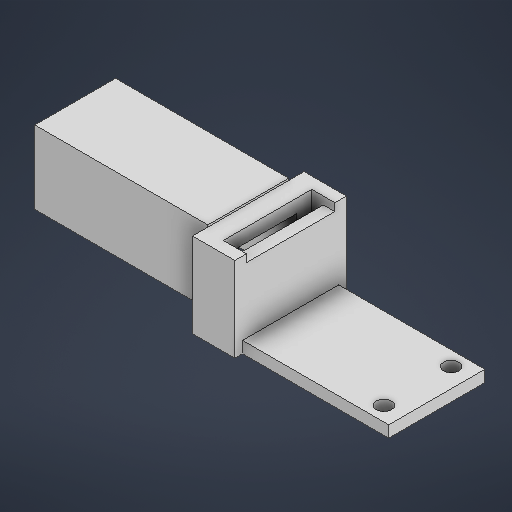
# Autodesk Inventor part: rgb-holder-group2
Saved by Autodesk Inventor 2026.1 (Build 301233000, 233)
## iProperties
Created: 2026-03-11
Part Number: rgb-holder-group2
Material: Generic
Document SubType Name: Modeling
Designer: ba2032
Density: 1 g/cm^3
Appearance: Default
Author: ba2032
Autodesk Inventor part; units mm, degrees
ref_plane "YZ Plane" through (0, 0, 0) normal (1, 0, 0) x (0, 1, 0)
ref_plane "XZ Plane" through (0, 0, 0) normal (0, 1, 0) x (-1, 0, 0)
ref_plane "XY Plane" through (0, 0, 0) normal (0, 0, 1) x (1, 0, 0)
sketch "Sketch1" plane through (0, 0, 0) normal (0, 1, 0) x (-1, 0, 0)
  line L0 (-20, 12.5) -> (20, 12.5)
  line L1 (20, 12.5) -> (20, -12.5)
  line L2 (20, -12.5) -> (-20, -12.5)
  line L3 (-20, -12.5) -> (-20, 12.5)
  line L4 (-20, 12.5) -> (20, -12.5) construction
  line L5 (20, 12.5) -> (-20, -12.5) construction
  circle A0 centre (-15, 8.75) radius 2
  circle A1 centre (-15, -8.75) radius 2
  point P0 (0, 0)
  dimension "d0" = 40
  dimension "d1" = 25
  dimension "d2" = 4
  dimension "d3" = 4
  constraints: 12 end point, 2 centre point, 2 midpoint, 2 parallel, 1 horizontal, 1 perpendicular
  measures "d0" distance of L1.end L2.end
  measures "d1" distance of L0.end L1.end
  measures "d2" diameter of A0
  measures "d3" diameter of A1
extrude "Extrusion1" add sketch "Sketch1" along normal blind 3 contours L0 L1 L2 L3 | A1
extrude "Extrusion2" cut sketch "Sketch1" along normal blind 3 contours A0 | A1
sketch "Sketch3" plane through (-20, 0, -12.5) normal (-1, 0, 0) x (0, 0, 1)
  line L0 (0, 0) -> (25, 0) projected
  line L1 (0, 0) -> (25, 0)
  line L2 (25, 0) -> (25, 22)
  line L3 (25, 22) -> (0, 22)
  line L4 (0, 22) -> (0, 0)
  point P0 (12.5, 0)
  dimension "d14" = 22
  constraints: 8 end point, 2 parallel, 1 horizontal, 1 perpendicular
  measures "d14" distance of L2.end L0.end
extrude "Extrusion4" add sketch "Sketch3" along normal blind 9
sketch "Sketch4" plane through (-20, 22, 12.5) normal (0, 1, 0) x (1, 0, 0)
  line L0 (-4, 24) -> (-1, 24)
  line L1 (-1, 24) -> (-1, 1)
  line L2 (-1, 1) -> (-4, 1)
  line L3 (-4, 1) -> (-4, 24)
  point P0 (20, 12.5)
  dimension "d17" = 3
  dimension "d18" = 23
  constraints: 8 end point, 2 parallel, 1 horizontal, 1 perpendicular
  measures "d17" distance of L0.start L0.end
  measures "d18" distance of L0.end L1.end
extrude "Extrusion5" cut sketch "Sketch4" against normal blind 21
sketch "Sketch6" plane through (-21, 22, -11.5) normal (-1, 0, 0) x (0, 0, 1)
  line L0 (0, 0) -> (23, 0) projected
  line L1 (0, 0) -> (23, 0)
  line L2 (23, 0) -> (23, -2)
  line L3 (23, -2) -> (0, -2)
  line L4 (0, -2) -> (0, 0)
  point P0 (11.5, -22)
  dimension "d26" = 2
  constraints: 8 end point, 2 parallel, 1 horizontal, 1 perpendicular
  measures "d26" distance of L0.end L2.end
extrude "Extrusion7" cut sketch "Sketch6" against normal blind 3
sketch "Sketch5" plane through (-29, 0, -12.5) normal (-1, 0, 0) x (0, 0, 1)
  line L0 (20, 18.5) -> (20, 3.5)
  line L1 (20, 3.5) -> (5, 3.5)
  line L2 (5, 3.5) -> (5, 18.5)
  line L3 (5, 18.5) -> (20, 18.5)
  point P0 (12.5, 0)
  dimension "d21" = 15
  dimension "d22" = 15
  constraints: 8 end point, 2 parallel, 1 perpendicular, 1 vertical
  measures "d21" distance of L0.start L0.end
  measures "d22" distance of L0.end L1.end
extrude "Extrusion6" cut sketch "Sketch5" against normal blind 10
sketch "Sketch7" plane through (-29, 0, -12.5) normal (-1, 0, 0) x (0, 0, 1)
  line L0 (20, 3.5) -> (5, 3.5) projected
  line L1 (5, 3.5) -> (2, 3.5)
  line L2 (2, 3.5) -> (2, 22.5)
  line L3 (2, 22.5) -> (5, 22.5)
  line L4 (5, 22.5) -> (5, 3.5)
  line L5 (5, 22.5) -> (20, 22.5)
  line L6 (20, 22.5) -> (20, 18.5)
  line L7 (20, 18.5) -> (5, 18.5)
  line L8 (5, 18.5) -> (5, 22.5)
  line L9 (20, 3.5) -> (20, 22.5)
  line L10 (20, 22.5) -> (23, 22.5)
  line L11 (23, 22.5) -> (23, 3.5)
  line L12 (23, 3.5) -> (20, 3.5)
  line L13 (25, 0) -> (25, 22) projected
  point P0 (12.5, 0)
  dimension "d29" = 3
  dimension "d30" = 19
  dimension "d31" = 15
  dimension "d32" = 3
  constraints: 24 end point, 6 parallel, 3 perpendicular, 1 horizontal, 1 point on line
  measures "d29" distance of L0.end L1.end
  measures "d30" distance of L1.end L2.end
  measures "d31" distance of L3.end L5.end
  measures "d32" distance of L5.end L10.end
extrude "Extrusion8" add sketch "Sketch7" along normal blind 1 contours L1 L2 L3 L4
extrude "Extrusion9" add sketch "Sketch7" along normal blind 45 contours L9 L6 L10 L11 L12 | L7 L4 L5 L6
extrude "Extrusion10" add sketch "Sketch7" along normal blind 45 contours L1 L2 L3 L4
sketch "Sketch8" plane through (20, 0, 12.5) normal (0, 0, 1) x (1, 0, 0)
  line L0 (-40, 22) -> (-49, 22) projected
  line L1 (-49, 22) -> (-40, 22)
  line L2 (-40, 22) -> (-40, 0)
  line L3 (-40, 0) -> (-49, 0)
  line L4 (-49, 0) -> (-49, 22)
  point P0 (-20, 0)
  constraints: 8 end point, 3 equal length, 1 perpendicular
extrude "Extrusion11" add sketch "Sketch8" along normal blind 2
sketch "Sketch9" plane through (20, 0, -12.5) normal (0, 0, -1) x (-1, 0, 0)
  line L0 (40, 22) -> (44, 22) projected
  line L1 (49, 22) -> (40, 22)
  line L2 (40, 22) -> (40, 0)
  line L3 (40, 0) -> (49, 0)
  line L4 (49, 0) -> (49, 22)
  point P0 (20, 0)
  constraints: 8 end point, 2 parallel, 1 horizontal, 1 perpendicular
extrude "Extrusion12" add sketch "Sketch9" along normal blind 2
sketch "Sketch10" plane through (-20, 0, -12.5) normal (1, 0, 0) x (0, 0, -1)
  line L0 (-27, 0) -> (-27, 22) projected
  line L1 (2, 22) -> (2, 0) projected
  line L2 (-27, 22) -> (2, 22)
  line L3 (2, 22) -> (2, 0)
  line L4 (2, 0) -> (-27, 0)
  line L5 (-27, 0) -> (-27, 22)
  point P0 (-12.5, 0)
  constraints: 8 end point, 2 parallel, 1 horizontal, 1 perpendicular
extrude "Extrusion13" add sketch "Sketch10" along normal blind 2
sketch "Sketch11" plane through (-20, 0, -12.5) normal (-1, 0, 0) x (0, 0, 1)
  line L0 (1, 22) -> (1, 20) projected
  line L1 (1, 22) -> (24, 22) projected
  line L2 (1, 20) -> (1, 22)
  line L3 (1, 22) -> (24, 22)
  line L4 (24, 22) -> (24, 20)
  line L5 (24, 20) -> (1, 20)
  point P0 (12.5, 0)
  constraints: 8 end point, 2 parallel, 1 perpendicular, 1 vertical
extrude "Extrusion14" cut sketch "Sketch11" against normal blind 2
body "Solid1"
